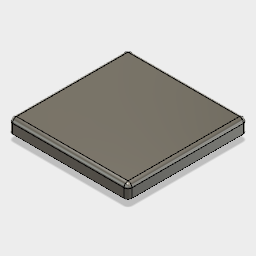
topbody v6 (Autodesk Fusion 360 design; units mm, degrees)
Autodesk Fusion 360 part; units mm, degrees
note: some values were not read from the file. Set by a fixed rule: which sketch regions a step uses.
sketch "Sketch1" plane through (0, 0, 0) normal (0, 1, 0) x (1, 0, 0)
  line L0 (0, 0) -> (89.803, 0)
  line L1 (89.803, 0) -> (89.803, 89.803)
  line L2 (89.803, 89.803) -> (0, 89.803)
  line L3 (0, 89.803) -> (0, 0)
  dimension "d1" = 89.803
  dimension "d2" = 89.803
  measures "d1" distance of L0.start L0.end
  measures "d2" distance of L0.start L2.end
extrude "Extrude1" add sketch "Sketch1" along normal blind 10 makes body 1
sketch "Sketch6" plane through (0, 0, 0) normal (0, -1, 0) x (1, 0, 0)
  line L0 (0, -89.803) -> (89.803, -89.803)
  line L1 (89.803, -89.803) -> (89.803, 0)
  line L2 (89.803, 0) -> (0, 0)
  line L3 (77.4015, -12.4015) -> (12.4015, -12.4015)
  line L4 (12.4015, -12.4015) -> (12.4015, -77.4015)
  line L5 (12.4015, -77.4015) -> (77.4015, -77.4015)
  line L6 (77.4015, -77.4015) -> (77.4015, -12.4015)
  line L7 (77.4015, -12.4015) -> (12.4015, -77.4015) construction
  line L8 (12.4015, -12.4015) -> (77.4015, -77.4015) construction
  point P0 (44.9015, -44.9015)
  dimension "d12" = 65
  dimension "d13" = 65
  measures "d12" distance of L3.end L4.end
  measures "d13" distance of L4.end L5.end
extrude "Extrude3" add sketch "Sketch6" against normal blind 1 bodies 1
fillet "Fillet2" radius 3 8 edges at (0, 5, 0) (44.9015, 10, 0) (0, 10, -44.9015) (89.803, 10, -44.9015) (44.9015, 10, -89.803) (89.803, 5, 0) (89.803, 5, -89.803) (0, 5, -89.803) on bodies 1
copy_body "Body->Comp2" bodies 1 removing the originals makes body 2 in component "topbody2"
sketch "Sketch7" plane through (0, 0, 0) normal (0, -1, 0) x (1, 0, 0)
  arc A0 (86.803, -89.803) -> (89.803, -86.803) centre (86.803, -86.803) ccw
  line L0 (89.803, -86.803) -> (89.803, -3)
  arc A1 (89.803, -3) -> (86.803, 0) centre (86.803, -3) ccw
  line L1 (86.803, 0) -> (3, 0)
  arc A2 (3, 0) -> (0, -3) centre (3, -3) ccw
  line L2 (0, -3) -> (0, -86.803)
  arc A3 (0, -86.803) -> (3, -89.803) centre (3, -86.803) ccw
  line L3 (3, -89.803) -> (86.803, -89.803)
  circle A4 centre (5, -5) radius 3
  circle A5 centre (5, -85) radius 3
  circle A6 centre (85, -85) radius 3
  circle A7 centre (85, -5) radius 3
  dimension "d17" = 6
  dimension "d18" = 6
  dimension "d19" = 6
  dimension "d20" = 6
  measures "d17" diameter of A4
  measures "d18" diameter of A5
  measures "d19" diameter of A6
  measures "d20" diameter of A7
extrude "Extrude1'" cut sketch "Sketch7" against normal blind 3 contours A4 | A5 | A6 | A7 bodies 2 in component "topbody2"
sketch "Sketch8" plane through (0, 0, 0) normal (0, -1, 0) x (1, 0, 0)
  circle A0 centre (85, -5) radius 3
  circle A1 centre (85, -85) radius 3
  circle A2 centre (5, -5) radius 3
  circle A3 centre (5, -85) radius 3
  arc A4 (86.803, -89.803) -> (89.803, -86.803) centre (86.803, -86.803) ccw
  line L0 (89.803, -86.803) -> (89.803, -3)
  arc A5 (89.803, -3) -> (86.803, 0) centre (86.803, -3) ccw
  line L1 (86.803, 0) -> (3, 0)
  arc A6 (3, 0) -> (0, -3) centre (3, -3) ccw
  line L2 (0, -3) -> (0, -86.803)
  arc A7 (0, -86.803) -> (3, -89.803) centre (3, -86.803) ccw
  line L3 (3, -89.803) -> (86.803, -89.803)
  line L4 (7.6, -15) -> (7.6, -75)
  line L5 (14.4179, -82.203) -> (69.8225, -82.203)
  line L6 (82.203, -71.2718) -> (82.203, -12.7891)
  line L7 (70, -7.6) -> (20, -7.6)
  line L8 (7.6, -15) -> (7.6, -7.6)
  line L9 (7.6, -7.6) -> (20, -7.6)
  line L10 (7.6, -7.6) -> (20, -7.6)
  line L11 (20, -7.6) -> (70, -7.6)
  line L12 (70, -7.6) -> (82.203, -7.6)
  line L13 (82.203, -12.7891) -> (82.203, -7.6)
  line L14 (82.203, -71.2718) -> (82.203, -82.203)
  line L15 (69.8225, -82.203) -> (82.203, -82.203)
  line L16 (14.4179, -82.203) -> (7.6, -82.203)
  line L17 (7.6, -75) -> (7.6, -82.203)
extrude "Extrude2" add sketch "Sketch8" along normal blind 5 contours L4 L5 L6 L7 L8 L9 L10 L11 L12 L13 L14 L15 L16 L17 bodies 2 in component "topbody2"
sketch "Sketch9" plane through (0, -5, 0) normal (0, -1, 0) x (1, 0, 0)
  line L0 (7.6, -7.6) -> (7.6, -82.203)
  line L1 (7.6, -82.203) -> (82.203, -82.203)
  line L2 (82.203, -82.203) -> (82.203, -7.6)
  line L3 (82.203, -7.6) -> (7.6, -7.6)
  line L4 (78.6515, -11.1515) -> (11.1515, -11.1515)
  line L5 (11.1515, -11.1515) -> (11.1515, -78.6515)
  line L6 (11.1515, -78.6515) -> (78.6515, -78.6515)
  line L7 (78.6515, -78.6515) -> (78.6515, -11.1515)
  line L8 (78.6515, -11.1515) -> (11.1515, -78.6515) construction
  line L9 (11.1515, -11.1515) -> (78.6515, -78.6515) construction
  point P0 (44.9015, -44.9015)
  dimension "d33" = 67.5
  dimension "d34" = 67.5
  measures "d33" distance of L5.end L6.end
  measures "d34" distance of L4.end L5.end
extrude "Extrude3'" cut sketch "Sketch9" against normal blind 10 contours L4 L5 L6 L7 bodies 2 in component "topbody2"
component "topbody2" placed x (1, 0, 0) y (0, 1, 0) z (0, 0, 1) at (0, 0, 0)
